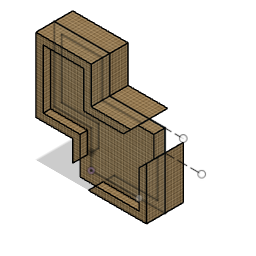
3d07 v12 (Autodesk Fusion 360 design; units mm, degrees)
Autodesk Fusion 360 part; units mm, degrees
sketch "Sketch1" plane through (0, 0, 0) normal (0, 0, 1) x (1, 0, 0)
  line L0 (0, 0) -> (40, 0)
  line L1 (40, 0) -> (40, 40)
  line L2 (40, 40) -> (10, 40)
  line L3 (0, 20) -> (0, 0)
  line L4 (-20, 60) -> (10, 60)
  line L5 (0, 20) -> (-20, 20)
  line L6 (-20, 20) -> (-20, 60)
  line L7 (-16, 56) -> (6, 56)
  line L8 (6, 56) -> (6, 36)
  line L9 (4, 24) -> (-16, 24)
  line L10 (-16, 24) -> (-16, 56)
  line L11 (6, 36) -> (27.5, 36)
  line L12 (36, 24.2786) -> (36, 4)
  line L13 (36, 4) -> (12.5, 4)
  line L14 (4, 12.5) -> (4, 24)
  line L15 (10, 60) -> (10, 40)
  line L16 (31.5, 40) -> (27.5, 36)
  line L17 (31.5, 40) -> (49.9198, 40) construction
  line L18 (40, 28.2786) -> (36, 24.2786)
  line L19 (40, 28.2786) -> (59.9507, 28.2786) construction
  line L20 (0, 8.5) -> (4, 12.5)
  line L21 (8.5, 0) -> (12.5, 4)
  line L22 (8.5, 0) -> (25.9429, 0) construction
  dimension "d1" = 40
  dimension "d3" = 30
  dimension "d4" = 40
  dimension "d5" = 30
  dimension "d6" = 60
  dimension "d7" = 22
  dimension "d8" = 32
  dimension "d9" = 4
  dimension "d10" = 4
  dimension "d13" = 4
  dimension "d14" = 4
  dimension "d18" = 4
  dimension "d19" = 90
  dimension "d20" = 90
  dimension "d21" = 32
  dimension "d22" = 32
  dimension "d23" = 135
  dimension "d24" = 135
  dimension "d26" = 45
  dimension "d27" = 12.0208
  dimension "d28" = 45
  dimension "d29" = 135
  dimension "d30" = 4
  dimension "d31" = 5.6569
  dimension "d32" = 45
  dimension "d33" = 45
  dimension "d34" = 2.2779
  dimension "d35" = 27.5
  dimension "d36" = 44.5477
  constraint horizontal L0
  constraint vertical L1
  constraint horizontal L2
  constraint vertical L3
  constraint coincident L0.start L3.end
  constraint horizontal L4
  constraint vertical L15
  constraint horizontal L5
  constraint vertical L6
  constraint horizontal L7
  constraint vertical L8
  constraint horizontal L9
  constraint vertical L10
  constraint horizontal L11
  constraint vertical L12
  constraint horizontal L13
  constraint vertical L14
  constraint coincident L3 L20.start
  constraint coincident L0 L21.start
  constraint coincident L2 L16.start
  constraint coincident L1 L18.start
  constraint horizontal L17
  constraint horizontal L19
  constraint horizontal L22
  measures "d1" distance of L0.start L0.end
  measures "d3" distance of L4.start L4.end
  measures "d4" distance of L4.start L5.end
  measures "d5" horizontal distance of L1.end L4.end
  measures "d6" vertical distance of L0.start L4.start
  measures "d7" distance of L7.start L7.end
  measures "d8" distance of L7.start L9.end
  measures "d9" distance of L6 L10
  measures "d10" distance of L5 L9
  measures "d13" distance of L3 L14
  measures "d14" distance of L0 L13
  measures "d18" distance of L2 L11
  measures "d19" angle of L11 L14
  measures "d20" angle of L11 L12
  measures "d21" distance of L11 L13
  measures "d22" distance of L12 L14
  measures "d23" angle of L16 L17
  measures "d24" angle of L18 L19
  measures "d26" angle of L21 L22
  measures "d27" distance of L20 L21
  measures "d28" angle of L12 L20
  measures "d29" angle of L0 L21
  measures "d30" vertical distance of L21.start L13.end
  measures "d31" distance of L21.start L13.end
  measures "d32" angle of L1 L16
  measures "d33" angle of L8 L18
  measures "d34" distance of L18 L21
  measures "d35" horizontal distance of L18.start L13.end
  measures "d36" distance of L20.start L16.start
extrude "Extrude2" add sketch "Sketch1" along normal blind 6 contours L0 L1 L2 L3 L7 L8 L9 L10 L11 L12 L13 L14 L16 L18 L20 L21 makes body 1
extrude "Extrude1" add sketch "Sketch1" along normal mid plane 20 separate body contours L0 L1 L12 L13 L18 L21 | L2 L3 L4 L5 L6 L7 L8 L9 L10 L11 L14 L15 L16 L20 makes body 2 at (-20, 33.3333, -3.3333) makes body 3 at (29.5, 0, 3.3333)
sketch "Sketch2" plane through (0, 0, 0) normal (0, 0, 1) x (1, 0, 0)
